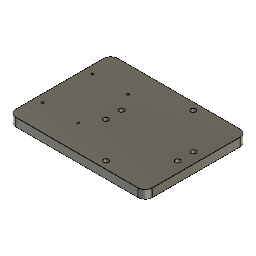
base v6 (Autodesk Fusion 360 design; units mm, degrees)
Autodesk Fusion 360 part; units mm, degrees
note: some values were not read from the file. Set by a fixed rule: which sketch regions a step uses.
sketch "Sketch1" plane through (0, 0, 0) normal (0, 0, 1) x (1, 0, 0)
  line L0 (10, 0) -> (182, 0)
  line L1 (192, 10) -> (192, 133.562)
  line L2 (182, 143.562) -> (10, 143.562)
  line L3 (0, 133.562) -> (0, 10)
  line L4 (126.5, 133.062) -> (126.5, 10.5)
  circle A0 centre (126.5, 133.062) radius 3.5
  circle A1 centre (126.5, 10.5) radius 3.5
  line L5 (126.5, 71.781) -> (192, 71.781)
  line L6 (177, 71.781) -> (76, 71.781)
  line L7 (76, 82.781) -> (76, 60.781)
  circle A2 centre (76, 82.781) radius 3.5
  circle A3 centre (76, 60.781) radius 3.5
  line L8 (177, 82.781) -> (177, 60.781)
  circle A4 centre (177, 82.781) radius 3.5
  circle A5 centre (177, 60.781) radius 3.5
  line L9 (11, 106.781) -> (61, 106.781)
  line L10 (61, 106.781) -> (61, 36.781)
  line L11 (61, 36.781) -> (11, 36.781)
  line L12 (11, 36.781) -> (11, 106.781)
  line L13 (11, 71.781) -> (0, 71.781)
  circle A6 centre (61, 106.781) radius 1.55
  circle A7 centre (11, 106.781) radius 1.55
  circle A8 centre (11, 36.781) radius 1.55
  circle A9 centre (61, 36.781) radius 1.55
  arc A10 (10, 143.562) -> (0, 133.562) centre (10, 133.562) ccw
  arc A11 (192, 133.562) -> (182, 143.562) centre (182, 133.562) ccw
  arc A12 (182, 0) -> (192, 10) centre (182, 10) ccw
  arc A13 (0, 10) -> (10, 0) centre (10, 10) ccw
  point P0 (192, 0)
  point P1 (192, 143.562)
  point P2 (76, 71.781)
  point P3 (126.5, 71.781)
  dimension "d1" = 143.562
  dimension "d3" = 7
  dimension "d4" = 7
  dimension "d5" = 122.562
  dimension "d6" = 90
  dimension "d7" = 101
  dimension "d8" = 22
  dimension "d9" = 7
  dimension "d10" = 7
  dimension "d11" = 15
  dimension "d12" = 50
  dimension "d13" = 70
  dimension "d14" = 15
  dimension "d15" = 90
  dimension "d16" = 3.1
  dimension "d17" = 3.1
  dimension "d18" = 3.1
  dimension "d19" = 3.1
  dimension "d20" = 10
  dimension "d21" = 10
  dimension "d22" = 10
  dimension "d23" = 10
  dimension "d42" = 11
  constraint horizontal L0
  constraint vertical L1
  constraint horizontal L2
  constraint vertical L3
  constraint vertical L4
  constraint coincident L4.start A0.centre
  constraint coincident L4.end A1.centre
  constraint midpoint L4 P3
  constraint perpendicular L4 L6
  constraint perpendicular L6 L7
  constraint midpoint L7 P2
  constraint coincident P2 L6.end
  constraint coincident L7.start A2.centre
  constraint coincident L7.end A3.centre
  constraint midpoint L6 P3
  constraint coincident P3 L5.start
  constraint symmetric L4 L7.start L8.start
  constraint symmetric L4 L7.end L8.end
  constraint symmetric L4 A2 A4
  constraint symmetric L4 A3 A5
  constraint horizontal L9
  constraint vertical L10
  constraint horizontal L11
  constraint vertical L12
  constraint midpoint L12 L13.start
  constraint coincident L9.end L10.start
  constraint coincident L9.start L12.end
  constraint coincident L11.end L12.start
  constraint coincident L10.end L11.start
  constraint coincident L3 L13.end
  constraint tangent L2 A10
  constraint tangent L3 A10
  constraint coincident L1 L5.end
  constraint coincident P1 L1
  constraint coincident P1 L2
  constraint tangent L1 A11
  constraint tangent L2 A11
  constraint coincident P0 L0
  constraint coincident P0 L1
  constraint tangent L0 A12
  constraint tangent L1 A12
  constraint tangent L0 A13
  constraint tangent L3 A13
  measures "d1" distance of P0 P1
  measures "d3" diameter of A0
  measures "d4" diameter of A1
  measures "d5" distance of L4.start L4.end
  measures "d6" angle of L1 L5
  measures "d7" distance of L6.start P2
  measures "d8" distance of L7.start L7.end
  measures "d9" diameter of A2
  measures "d10" diameter of A3
  measures "d11" distance of L1 L8
  measures "d12" distance of L9.start L9.end
  measures "d13" distance of L9.start L11.end
  measures "d14" distance of L7 L10
  measures "d15" angle of L3 L13
  measures "d16" diameter of A6
  measures "d17" diameter of A7
  measures "d18" diameter of A8
  measures "d19" diameter of A9
  measures "d20" radius of A10
  measures "d21" radius of A11
  measures "d22" radius of A12
  measures "d23" radius of A13
  measures "d42" distance of L13.start L13.end
extrude "Extrude1" add sketch "Sketch1" along normal blind 10 contours L0 L1 L2 L3 A10 A11 A12 A13 | L9 L10 L11 L12 A6 A7 A8 A9
extrude "Extrude2" add 1 faces at (126.5014, 98.4319, 10) along direction (0, 0, 1) blind 1
extrude "Extrude3" add 1 faces at (32.1961, 68.4582, 0) along direction (0, 0, -1) blind 1
equation "d7 = 90 mm + 11 mm"
